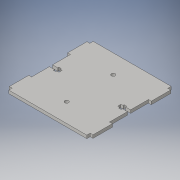
# Autodesk Inventor part: MountBase
Saved by Autodesk Inventor 2016 (Build 200138000, 138)
## iProperties
Created: 2016-07-10
Part Number: MountBase
Material: Generic
Document SubType Name: Modeling
Designer: jeffkub
Density: 1 g/cm^3
Appearance: Default
Author: jeffkub
Autodesk Inventor part; units mm, degrees
ref_plane "YZ Plane" through (0, 0, 0) normal (1, 0, 0) x (0, 1, 0)
ref_plane "XZ Plane" through (0, 0, 0) normal (0, 1, 0) x (-1, 0, 0)
ref_plane "XY Plane" through (0, 0, 0) normal (0, 0, 1) x (1, 0, 0)
sketch "Sketch1" plane through (0, 0, 0) normal (0, 1, 0) x (-1, 0, 0)
  line L0 (38.2, 41.375) -> (0, 41.375)
  line L1 (0, -41.375) -> (38.2, -41.375)
  line L2 (38.2, -41.375) -> (38.2, -38.1)
  line L3 (38.2, 41.375) -> (-38.2, -41.375) construction
  line L4 (-38.2, 41.375) -> (38.2, -41.375) construction
  line L5 (38.2, -38.1) -> (41, -38.1)
  line L6 (41, -38.1) -> (41, -19.05)
  line L7 (41, 38.1) -> (38.2, 38.1)
  line L8 (41, -19.05) -> (38.2, -19.05)
  line L9 (41, 19.05) -> (38.2, 19.05)
  line L10 (0, -57.1711) -> (0, 53.4379)
  line L11 (38.2, -38.1) -> (38.2, -19.05) construction
  line L12 (38.2, -19.05) -> (38.2, -1.55)
  line L13 (38.2, 19.05) -> (38.2, 38.1) construction
  line L14 (38.2, 38.1) -> (38.2, 41.375)
  line L15 (41, 19.05) -> (41, 38.1)
  line L16 (41, -19.05) -> (41, 19.05) construction
  line L17 (43.0653, 0) -> (18.1238, 0)
  line L18 (38.2, 1.55) -> (33.2, 1.55)
  line L19 (33.2, 1.55) -> (33.2, 2.1343)
  line L20 (33.2, 2.7) -> (32.6343, 2.7) construction
  line L21 (30.8, 2.7) -> (30.8, 1.55)
  line L22 (30.8, 1.55) -> (28.8, 1.55)
  line L23 (28.8, 1.55) -> (28.8, 0)
  arc A0 (33.2, 2.1343) -> (32.6343, 2.7) centre (32.9172, 2.4172) ccw
  line L24 (33.2, 2.1343) -> (33.2, 2.7) construction
  line L25 (32.6343, 2.7) -> (30.8, 2.7)
  line L26 (38.2, -1.55) -> (33.2, -1.55)
  line L27 (33.2, -1.55) -> (33.2, -2.1343)
  line L28 (30.8, -2.7) -> (30.8, -1.55)
  line L29 (30.8, -1.55) -> (28.8, -1.55)
  line L30 (28.8, -1.55) -> (28.8, 0)
  arc A1 (32.6343, -2.7) -> (33.2, -2.1343) centre (32.9172, -2.4172) ccw
  line L31 (32.6343, -2.7) -> (30.8, -2.7)
  line L32 (38.2, -1.55) -> (38.2, 1.55) construction
  line L33 (38.2, 1.55) -> (38.2, 19.05)
  line L34 (-38.2, 41.375) -> (0, 41.375)
  line L35 (0, -41.375) -> (-38.2, -41.375)
  line L36 (-38.2, -41.375) -> (-38.2, -38.1)
  line L37 (-38.2, -38.1) -> (-41, -38.1)
  line L38 (-41, -38.1) -> (-41, -19.05)
  line L39 (-41, 38.1) -> (-38.2, 38.1)
  line L40 (-41, -19.05) -> (-38.2, -19.05)
  line L41 (-41, 19.05) -> (-38.2, 19.05)
  line L42 (-38.2, -19.05) -> (-38.2, -1.55)
  line L43 (-38.2, 38.1) -> (-38.2, 41.375)
  line L44 (-41, 19.05) -> (-41, 38.1)
  line L45 (-38.2, 1.55) -> (-33.2, 1.55)
  line L46 (-33.2, 1.55) -> (-33.2, 2.1343)
  line L47 (-30.8, 2.7) -> (-30.8, 1.55)
  line L48 (-30.8, 1.55) -> (-28.8, 1.55)
  line L49 (-28.8, 1.55) -> (-28.8, 0)
  arc A2 (-32.6343, 2.7) -> (-33.2, 2.1343) centre (-32.9172, 2.4172) ccw
  line L50 (-32.6343, 2.7) -> (-30.8, 2.7)
  line L51 (-38.2, -1.55) -> (-33.2, -1.55)
  line L52 (-33.2, -1.55) -> (-33.2, -2.1343)
  arc A3 (-33.2, -2.1343) -> (-32.6343, -2.7) centre (-32.9172, -2.4172) ccw
  line L53 (-30.8, -2.7) -> (-30.8, -1.55)
  line L54 (-30.8, -1.55) -> (-28.8, -1.55)
  line L55 (-28.8, -1.55) -> (-28.8, 0)
  line L56 (-38.2, 1.55) -> (-38.2, 19.05)
  line L57 (-32.6343, -2.7) -> (-30.8, -2.7)
  point P0 (0, 0)
  point P1 (0, 0)
  dimension "d0" = 76.4
  dimension "d2" = 76.2
  dimension "d3" = 2.8
  dimension "d4" = 19.05
  dimension "d5" = 82.75
  dimension "d6" = 3.1
  dimension "d7" = 5
  dimension "d8" = 0.4
  dimension "d9" = 2.4
  dimension "d10" = 5.4
  dimension "d11" = 2
  constraints: 116 end point, 40 perpendicular, 33 symmetric about line, 27 point on line, 9 point on circle, 4 centre point, 4 equal length, 4 vertical, 3 horizontal, 3 midpoint, 1 parallel, 3 other
  measures "d0" distance of L0.start L4.start
  measures "d2" distance between parallel lines of L7 L5
  measures "d3" distance between parallel lines of L6 L11
  measures "d4" distance of L5.end L6.end
  measures "d5" distance between parallel lines of L0 L1
  measures "d6" diameter of L18 L17
  measures "d7" distance between parallel lines of L12 L19
  measures "d8" radius of A0
  measures "d9" distance between parallel lines of L21 L19
  measures "d10" diameter of L25 L17
  measures "d11" distance of L21.end L22.end
extrude "Extrusion1" add sketch "Sketch1" along normal blind 3
sketch "Sketch2" plane through (0, 0, 0) normal (0, -1, 0) x (1, 0, 0)
  circle A0 centre (0, -22.86) radius 16 construction
  circle A1 centre (0, 22.86) radius 16 construction
  circle A2 centre (0, -22.86) radius 1.8844
  circle A3 centre (0, 22.86) radius 1.8844
  point P0 (0, 0)
  dimension "d14" = 32
  dimension "d15" = 22.86
  dimension "d16" = 22.86
  dimension "d17" = 3.7687
  constraints: 4 centre point, 2 coincident, 2 equal radius, 2 vertical alignment
  measures "d14" diameter of A0
  measures "d15" distance of point (0, 0) A0.centre
  measures "d16" distance of point (0, 0) A1.centre
  measures "d17" diameter of A2
extrude "Extrusion2" cut sketch "Sketch2" against normal through all
equation "\"d16\" = d15"
body "Solid1"
